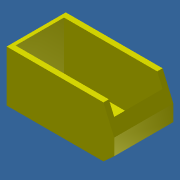
# Autodesk Inventor part: bin
Saved by Autodesk Inventor 2012 (Build 160160000, 160)
## iProperties
Created: 2012-11-30
Part Number: bin
Material: Thermoplastic Resin
Document SubType Name: Modeling
Designer: Ed
Mass: 4368.56 g
Surface Area: 5272.35 cm^2
Volume: 3412.93 cm^3
Density: 1.28 g/cm^3
Author: Ed
Autodesk Inventor part; units mm, degrees
note: some values were not read from the file. Chosen so that the rebuilt part matches the saved one: direction of "Hole1".
ref_plane "YZ Plane" through (0, 0, 0) normal (1, 0, 0) x (0, 1, 0)
ref_plane "XZ Plane" through (0, 0, 0) normal (0, 1, 0) x (-1, 0, 0)
ref_plane "XY Plane" through (0, 0, 0) normal (0, 0, 1) x (1, 0, 0)
sketch "Sketch1" plane through (0, 0, 0) normal (0, 0, 1) x (1, 0, 0)
  line L0 (0, 0) -> (342.9, 0)
  line L1 (342.9, 0) -> (342.9, -180.975)
  line L2 (342.9, -180.975) -> (0, -180.975)
  line L3 (0, -180.975) -> (0, 0)
  line L4 (342.9, -88.9) -> (381, -88.9)
  line L5 (381, -88.9) -> (381, -146.05)
  line L6 (381, -146.05) -> (342.9, -146.05)
  line L7 (342.9, -146.05) -> (342.9, -88.9)
  line L8 (381, -146.05) -> (342.9, -180.975)
  line L9 (381, -88.9) -> (342.9, 0)
  dimension "d0" = 342.9
  dimension "d1" = 180.975
  dimension "d2" = 88.9
  dimension "d3" = 34.925
  dimension "d4" = 38.1
  constraints: 20 end point, 4 parallel, 2 horizontal, 2 perpendicular, 1 point on line
  measures "d0" distance of L1.end L2.end
  measures "d1" distance of L2.end L0.start
  measures "d2" vertical distance of L4.end L0.end
  measures "d3" vertical distance of L5.end L1.end
  measures "d4" distance of L4.start L4.end
extrude "Extrusion1" add sketch "Sketch1" along normal blind 209.55
shell "Shell1" thickness 19.05 removed faces 2 at (228.6, 0, 69.85) at (355.6, -29.6333, 139.7) ; own thickness 19.05 on faces at (114.3, -60.325, 209.55) (381, -127, 69.85) (114.3, -60.325, 0) ; own thickness 12.7 on faces at (0, -60.325, 69.85) ; own thickness 3.175 on faces at (114.3, -180.975, 69.85) (355.6, -169.3333, 69.85)
hole "Hole1" at (0, -63.5, 166.6875) direction (1, 0, 0) diameter 11.1125 end up to surface
body "Solid1"
